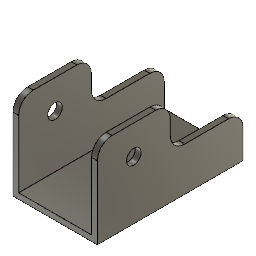
CUERPO UNIDO v3 (Autodesk Fusion 360 archive; units mm, degrees)
design "BASE"
Autodesk Fusion 360 part; units mm, degrees
sketch "Boceto1" plane through (0, 0, 0) normal (0, 0, 1) x (1, 0, 0)
  line L0 (0, 0) -> (0, 50)
  line L1 (0, 0) -> (0, -50)
  line L2 (0, 50) -> (58, 50)
  line L3 (58, 50) -> (58, -50)
  line L4 (58, -50) -> (0, -50)
  constraint coincident L0.start L1.start
  constraint vertical L0
  constraint parallel L0 L1
  constraint perpendicular L1 L2
  constraint perpendicular L2 L3
  constraint perpendicular L3 L4
extrude "Extruir1" add sketch "Boceto1" along normal blind 4 makes body 1
sketch "Boceto2" plane through (0, 0, 0) normal (0, 1, 0) x (1, 0, 0)
sketch "Boceto3" plane through (58, 0, 0) normal (1, 0, 0) x (0, 1, 0)
  line L0 (-50, 0) -> (50, 0)
  line L1 (50, 0) -> (50, 4)
  line L2 (50, 4) -> (-50, 4)
  line L3 (-50, 4) -> (-50, 0)
  line L4 (-50, 4) -> (-50, 50)
  line L5 (50, 4) -> (50, 20)
  line L6 (-40, 60) -> (-10, 60)
  line L7 (0, 50) -> (0, 40)
  line L8 (10, 30) -> (40, 30)
  arc A0 (-40, 60) -> (-50, 50) centre (-40, 50) ccw
  arc A1 (0, 50) -> (-10, 60) centre (-10, 50) ccw
  arc A2 (0, 40) -> (10, 30) centre (10, 40) ccw
  arc A3 (50, 20) -> (40, 30) centre (40, 20) ccw
  circle A4 centre (-25, 40) radius 5
  dimension "d8" = 10
  dimension "d9" = 10
  constraint coincident L2.end L3.start
  constraint perpendicular L2 L4
  constraint coincident L1.end L2.start
  constraint perpendicular L2 L5
  constraint perpendicular L4 L6
  constraint perpendicular L6 L7
  constraint perpendicular L5 L8
  constraint tangent L6 A0
  constraint tangent L4 A0
  constraint tangent L6 A1
  constraint tangent L7 A1
  constraint tangent L7 A2
  constraint tangent L8 A2
  constraint equal A1 A2
  constraint tangent L8 A3
  constraint tangent L5 A3
  constraint equal A1 A3
  measures "d8" radius of A0
  measures "d9" radius of A1
extrude "Extruir2" add sketch "Boceto3" against normal blind 4 contours L2 L4 L5 L6 L7 L8 A0 A1 A2 A3 | A4 bodies 1
extrude "Extruir3" cut sketch "Boceto3" against normal blind 15 contours A4 bodies 1
split "Dividir1" by plane through (0, 0, 4) normal (0, 0, 1) bodies 1 makes body 2 at (54, 2.859, 12.7006)
copy_body "CopiarPegarCuerpos1" bodies 2 makes body 3
move_body "Desplazar1" bodies 3 to x (1, 0, 0) y (0, 1, 0) z (0, 0, 1) at (-54, 0, 0)
combine "Combinar1" operation add target body 2 tool bodies 3 1

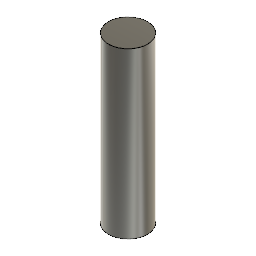
design "CILINDRO DE UNION"
Autodesk Fusion 360 part; units mm, degrees
cylinder "CilindroPrimitivo1" add diameter 10 height 42 placed x (1, 0, 0) y (0, 1, 0) z (0, 0, 1) at (0, 0, 0)

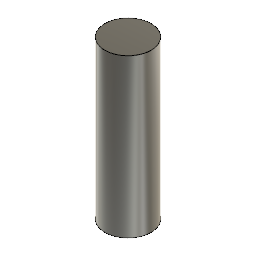
design "CILINDRO UNION ANTEBRAZO"
Autodesk Fusion 360 part; units mm, degrees
cylinder "CilindroPrimitivo1" add diameter 10 height 34 placed x (1, 0, 0) y (0, 1, 0) z (0, 0, 1) at (0, 0, 0)

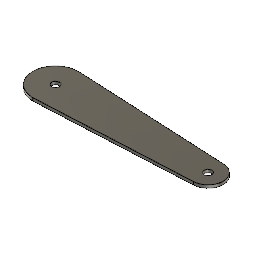
design "ANTEBRAZO"
Autodesk Fusion 360 part; units mm, degrees
sketch "Boceto1" plane through (0, 0, 0) normal (0, 0, 1) x (1, 0, 0)
  circle A0 centre (0, 0) radius 30
  circle A1 centre (200, 0) radius 20
  line L0 (-0.0033, 30) -> (200.9963, 19.9752)
  line L1 (200.9963, -19.9752) -> (-0.0033, -30)
  circle A2 centre (0, 0) radius 5
  circle A3 centre (200, 0) radius 5
  constraint coincident A0.centre A2.centre
  constraint coincident A0 L0.start
  constraint coincident A1 L0.end
  constraint tangent A1 L0
  constraint coincident A1 L1.start
  constraint coincident A0 L1.end
  constraint tangent A1 L1
  constraint concentric A0 A2
  constraint concentric A1 A3
extrude "Extruir1" add sketch "Boceto1" along normal blind 4 contours A0 L0 L1 | A0 A1 L0 L1 | A1
sketch "Boceto2" plane through (0, 0, 4) normal (0, 0, 1) x (-1, 0, 0)
  circle A0 centre (-200, 0) radius 5
  circle A1 centre (0, 0) radius 5
  arc A2 (0.0033, -30) -> (0.0033, 30) centre (0, 0) ccw
  line L0 (0.0033, 30) -> (-200.9963, 19.9752)
  arc A3 (-200.9963, 19.9752) -> (-200.9963, -19.9752) centre (-200, 0) ccw
  line L1 (-200.9963, -19.9752) -> (0.0033, -30)
  line L2 (0, 0) -> (-40, 0)
  line L3 (-40, 0) -> (-80, 0)
  line L4 (-80, 0) -> (-120, 0)
  line L5 (-120, 0) -> (-160, 0)
  line L6 (-160, 0) -> (-200, 0)
  line L7 (0, 0) -> (15, 0)
  constraint coincident A1.centre A2.centre
  constraint horizontal L2
  constraint parallel L2 L3
  constraint parallel L3 L4
  constraint parallel L2 L7

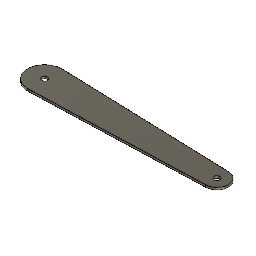
design "BRAZO"
Autodesk Fusion 360 part; units mm, degrees
sketch "Boceto1" plane through (0, 0, 0) normal (0, 0, 1) x (1, 0, 0)
  circle A0 centre (0, 0) radius 30
  circle A1 centre (300, 0) radius 20
  line L0 (-0.001, 30) -> (300.6656, 19.9889)
  line L1 (300, -20) -> (1.0011, -29.9833)
  circle A2 centre (300, 0) radius 5
  circle A3 centre (0, 0) radius 5
  line L2 (0, 0) -> (50, 0)
  line L3 (50, 0) -> (100, 0)
  line L4 (150, 0) -> (200, 0)
  line L5 (100, 0) -> (150, 0)
  line L6 (250, 0) -> (300, 0)
  line L7 (200, 0) -> (250, 0)
  line L8 (0, 0) -> (-15, 0)
  constraint coincident A0.centre A3.centre
  constraint coincident A0 L0.start
  constraint coincident A1 L0.end
  constraint tangent A1 L0
  constraint coincident A1 L1.start
  constraint coincident A0 L1.end
  constraint tangent A0 L1
  constraint concentric A1 A2
  constraint horizontal L2
  constraint parallel L2 L3
  constraint horizontal L5
  constraint parallel L4 L5
  constraint horizontal L7
  constraint parallel L6 L7
  constraint horizontal L8
extrude "Extruir2" add sketch "Boceto1" along normal blind 4 contours A0 L0 | A0 A1 L1 L2 L3 L4 L5 L6 L7 | A0 A1 L0 L2 L3 L4 L5 L6 L7 | A1 picked at (-1.5634, 21.558)
extrude "Extruir1" [suppressed]
